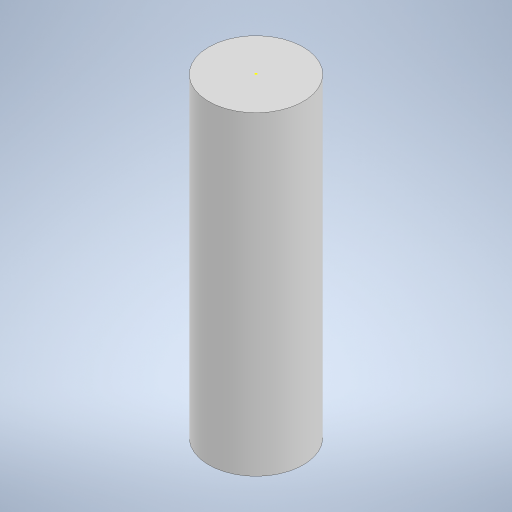
# Autodesk Inventor part: tale inner
Saved by Autodesk Inventor 2023 (Build 270158000, 158)
## iProperties
Created: 2022-10-23
Part Number: tale inner
Material: 一般
Document SubType Name: Modeling
Designer: ellie
Density: 1 g/cm^3
Appearance: 既定
Author: ellie
Autodesk Inventor part; units mm, degrees
ref_plane "YZ Plane" through (0, 0, 0) normal (1, 0, 0) x (0, 1, 0)
ref_plane "XZ Plane" through (0, 0, 0) normal (0, 1, 0) x (-1, 0, 0)
ref_plane "XY Plane" through (0, 0, 0) normal (0, 0, 1) x (1, 0, 0)
sketch "スケッチ1" plane through (0, 0, 0) normal (0, 1, 0) x (-1, 0, 0)
  circle A0 centre (0, 0) radius 2.25
  dimension "d0" = 4.5
  constraints: 1 centre point, 1 coincident
  measures "d0" diameter of A0
extrude "押し出し1" add sketch "スケッチ1" along normal blind 15
sketch "スケッチ2" plane through (0, 15, 0) normal (0, 1, 0) x (1, 0, 0)
  point P0 (0, 0)
